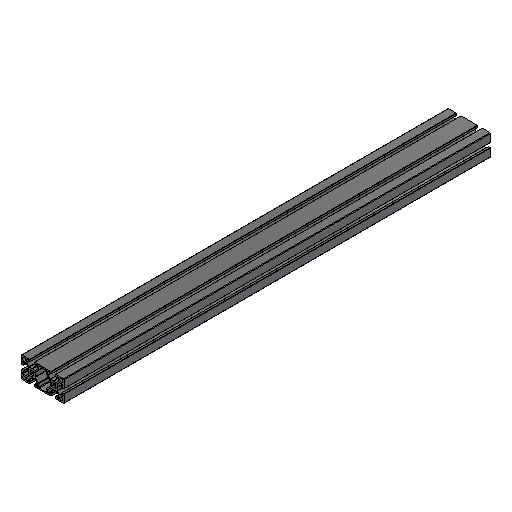
# Autodesk Inventor part: PROFILE
Saved by Autodesk Inventor 2022.5 (Build 265521000, 521)
## iProperties
Created: 2022-08-08
Part Number: PROFILE
Material: AL6061
Document SubType Name: Modeling
Designer: 박성규
Density: 2.7 g/cm^3
Description: 3
MAKER: DY PROFILE
DocNumber: DP 40X80-240L.ipt
Folder: 구매품\19. PIPE 형강류\AL PROFILE\DP TYPE\DP 40X80\
VDS_Category: 엔지니어링
Detail Description: Purchased products
Author: 최신영
Revision Number: B
Title: DP4080-802L
Autodesk Inventor part; units mm, degrees
ref_plane "YZ Plane" through (0, 0, 0) normal (1, 0, 0) x (0, 1, 0)
ref_plane "XZ Plane" through (0, 0, 0) normal (0, 1, 0) x (-1, 0, 0)
ref_plane "XY Plane" through (0, 0, 0) normal (0, 0, 1) x (1, 0, 0)
sketch "스케치3" plane through (0, 0, 0) normal (0, 0, 1) x (1, 0, 0)
  line L0 (0.0593, 17.8696) -> (6.8093, 17.8696)
  arc A0 (7.8093, 16.8696) -> (6.8093, 17.8696) centre (6.8093, 16.8696) ccw
  line L1 (7.8093, 16.8696) -> (7.8093, 10.9554)
  arc A1 (7.8093, 10.9554) -> (8.1022, 10.2483) centre (8.8093, 10.9554) ccw
  line L2 (8.1022, 10.2483) -> (14.2664, 4.0841)
  arc A2 (14.5593, 3.377) -> (14.2664, 4.0841) centre (13.5593, 3.377) ccw
  line L3 (14.5593, 3.377) -> (14.5593, -3.6377)
  arc A3 (14.2664, -4.3448) -> (14.5593, -3.6377) centre (13.5593, -3.6377) ccw
  line L4 (14.2664, -4.3448) -> (8.1022, -10.5091)
  arc A4 (8.1022, -10.5091) -> (7.8093, -11.2162) centre (8.8093, -11.2162) ccw
  line L5 (7.8093, -11.2162) -> (7.8093, -17.1304)
  arc A5 (6.8093, -18.1304) -> (7.8093, -17.1304) centre (6.8093, -17.1304) ccw
  line L6 (6.8093, -18.1304) -> (0.0593, -18.1304)
  line L7 (0.0593, -18.1304) -> (-6.6907, -18.1304)
  arc A6 (-7.6907, -17.1304) -> (-6.6907, -18.1304) centre (-6.6907, -17.1304) ccw
  line L8 (-7.6907, -17.1304) -> (-7.6907, -11.2162)
  arc A7 (-7.6907, -11.2162) -> (-7.9836, -10.5091) centre (-8.6907, -11.2162) ccw
  line L9 (-7.9836, -10.5091) -> (-14.1478, -4.3448)
  arc A8 (-14.4407, -3.6377) -> (-14.1478, -4.3448) centre (-13.4407, -3.6377) ccw
  line L10 (-14.4407, -3.6377) -> (-14.4407, 3.377)
  arc A9 (-14.1478, 4.0841) -> (-14.4407, 3.377) centre (-13.4407, 3.377) ccw
  line L11 (-14.1478, 4.0841) -> (-7.9836, 10.2483)
  arc A10 (-7.9836, 10.2483) -> (-7.6907, 10.9554) centre (-8.6907, 10.9554) ccw
  line L12 (-7.6907, 10.9554) -> (-7.6907, 16.8696)
  arc A11 (-6.6907, 17.8696) -> (-7.6907, 16.8696) centre (-6.6907, 16.8696) ccw
  line L13 (-6.6907, 17.8696) -> (0.0593, 17.8696)
  line L14 (39.0593, 19.8696) -> (24.7093, 19.8696)
  arc A12 (24.7093, 19.8696) -> (24.2093, 19.3696) centre (24.7093, 19.3696) ccw
  line L15 (24.2093, 19.3696) -> (24.2093, 16.1696)
  arc A13 (24.2093, 16.1696) -> (24.7093, 15.6696) centre (24.7093, 16.1696) ccw
  line L16 (24.7093, 15.6696) -> (26.6593, 15.6696)
  arc A14 (26.6593, 15.6696) -> (27.1593, 16.1696) centre (26.6593, 16.1696) ccw
  line L17 (27.1593, 16.1696) -> (27.1593, 17.3696)
  arc A15 (27.6593, 17.8696) -> (27.1593, 17.3696) centre (27.6593, 17.3696) ccw
  line L18 (27.6593, 17.8696) -> (29.8093, 17.8696)
  arc A16 (30.3093, 17.3696) -> (29.8093, 17.8696) centre (29.8093, 17.3696) ccw
  line L19 (30.3093, 17.3696) -> (30.3093, 12.061)
  arc A17 (30.1815, 11.7272) -> (30.3093, 12.061) centre (29.8093, 12.061) ccw
  line L20 (30.1815, 11.7272) -> (25.9734, 7.0358)
  arc A18 (25.6012, 6.8696) -> (25.9734, 7.0358) centre (25.6012, 7.3696) ccw
  line L21 (25.6012, 6.8696) -> (20.5593, 6.8696)
  line L22 (20.5593, 6.8696) -> (20.0593, 6.3696)
  line L23 (20.0593, 6.3696) -> (19.5593, 6.8696)
  line L24 (19.5593, 6.8696) -> (14.5174, 6.8696)
  arc A19 (14.1452, 7.0358) -> (14.5174, 6.8696) centre (14.5174, 7.3696) ccw
  line L25 (14.1452, 7.0358) -> (9.9371, 11.7272)
  arc A20 (9.8093, 12.061) -> (9.9371, 11.7272) centre (10.3093, 12.061) ccw
  line L26 (9.8093, 12.061) -> (9.8093, 17.3696)
  arc A21 (10.3093, 17.8696) -> (9.8093, 17.3696) centre (10.3093, 17.3696) ccw
  line L27 (10.3093, 17.8696) -> (12.4593, 17.8696)
  arc A22 (12.9593, 17.3696) -> (12.4593, 17.8696) centre (12.4593, 17.3696) ccw
  line L28 (12.9593, 17.3696) -> (12.9593, 16.1696)
  arc A23 (12.9593, 16.1696) -> (13.4593, 15.6696) centre (13.4593, 16.1696) ccw
  line L29 (13.4593, 15.6696) -> (15.4093, 15.6696)
  arc A24 (15.4093, 15.6696) -> (15.9093, 16.1696) centre (15.4093, 16.1696) ccw
  line L30 (15.9093, 16.1696) -> (15.9093, 19.3696)
  arc A25 (15.9093, 19.3696) -> (15.4093, 19.8696) centre (15.4093, 19.3696) ccw
  line L31 (15.4093, 19.8696) -> (-15.2907, 19.8696)
  arc A26 (-15.2907, 19.8696) -> (-15.7907, 19.3696) centre (-15.2907, 19.3696) ccw
  line L32 (-15.7907, 19.3696) -> (-15.7907, 16.1696)
  arc A27 (-15.7907, 16.1696) -> (-15.2907, 15.6696) centre (-15.2907, 16.1696) ccw
  line L33 (-15.2907, 15.6696) -> (-13.3407, 15.6696)
  arc A28 (-13.3407, 15.6696) -> (-12.8407, 16.1696) centre (-13.3407, 16.1696) ccw
  line L34 (-12.8407, 16.1696) -> (-12.8407, 17.3696)
  arc A29 (-12.3407, 17.8696) -> (-12.8407, 17.3696) centre (-12.3407, 17.3696) ccw
  line L35 (-12.3407, 17.8696) -> (-10.1907, 17.8696)
  arc A30 (-9.6907, 17.3696) -> (-10.1907, 17.8696) centre (-10.1907, 17.3696) ccw
  line L36 (-9.6907, 17.3696) -> (-9.6907, 11.8696)
  line L37 (-9.6907, 11.8696) -> (-14.1756, 6.8696)
  line L38 (-14.1756, 6.8696) -> (-19.4407, 6.8696)
  line L39 (-19.4407, 6.8696) -> (-19.9407, 6.3696)
  line L40 (-19.9407, 6.3696) -> (-20.4407, 6.8696)
  line L41 (-20.4407, 6.8696) -> (-25.4826, 6.8696)
  arc A31 (-25.8548, 7.0358) -> (-25.4826, 6.8696) centre (-25.4826, 7.3696) ccw
  line L42 (-25.8548, 7.0358) -> (-30.0629, 11.7272)
  arc A32 (-30.1907, 12.061) -> (-30.0629, 11.7272) centre (-29.6907, 12.061) ccw
  line L43 (-30.1907, 12.061) -> (-30.1907, 17.3696)
  arc A33 (-29.6907, 17.8696) -> (-30.1907, 17.3696) centre (-29.6907, 17.3696) ccw
  line L44 (-29.6907, 17.8696) -> (-27.5407, 17.8696)
  arc A34 (-27.0407, 17.3696) -> (-27.5407, 17.8696) centre (-27.5407, 17.3696) ccw
  line L45 (-27.0407, 17.3696) -> (-27.0407, 16.1696)
  arc A35 (-27.0407, 16.1696) -> (-26.5407, 15.6696) centre (-26.5407, 16.1696) ccw
  line L46 (-26.5407, 15.6696) -> (-24.5907, 15.6696)
  arc A36 (-24.5907, 15.6696) -> (-24.0907, 16.1696) centre (-24.5907, 16.1696) ccw
  line L47 (-24.0907, 16.1696) -> (-24.0907, 19.3696)
  arc A37 (-24.0907, 19.3696) -> (-24.5907, 19.8696) centre (-24.5907, 19.3696) ccw
  line L48 (-24.5907, 19.8696) -> (-38.9407, 19.8696)
  arc A38 (-38.9407, 19.8696) -> (-39.9407, 18.8696) centre (-38.9407, 18.8696) ccw
  line L49 (-39.9407, 18.8696) -> (-39.9407, 4.5196)
  arc A39 (-39.9407, 4.5196) -> (-39.4407, 4.0196) centre (-39.4407, 4.5196) ccw
  line L50 (-39.4407, 4.0196) -> (-36.2407, 4.0196)
  arc A40 (-36.2407, 4.0196) -> (-35.7407, 4.5196) centre (-36.2407, 4.5196) ccw
  line L51 (-35.7407, 4.5196) -> (-35.7407, 6.4696)
  arc A41 (-35.7407, 6.4696) -> (-36.2407, 6.9696) centre (-36.2407, 6.4696) ccw
  line L52 (-36.2407, 6.9696) -> (-37.4407, 6.9696)
  arc A42 (-37.9407, 7.4696) -> (-37.4407, 6.9696) centre (-37.4407, 7.4696) ccw
  line L53 (-37.9407, 7.4696) -> (-37.9407, 9.6196)
  arc A43 (-37.4407, 10.1196) -> (-37.9407, 9.6196) centre (-37.4407, 9.6196) ccw
  line L54 (-37.4407, 10.1196) -> (-32.1321, 10.1196)
  arc A44 (-31.7983, 9.9918) -> (-32.1321, 10.1196) centre (-32.1321, 9.6196) ccw
  line L55 (-31.7983, 9.9918) -> (-27.1069, 5.7837)
  arc A45 (-26.9407, 5.4115) -> (-27.1069, 5.7837) centre (-27.4407, 5.4115) ccw
  line L56 (-26.9407, 5.4115) -> (-26.9407, 0.3696)
  line L57 (-26.9407, 0.3696) -> (-26.4407, -0.1304)
  line L58 (-26.4407, -0.1304) -> (-26.9407, -0.6304)
  line L59 (-26.9407, -0.6304) -> (-26.9407, -5.6723)
  arc A46 (-27.1069, -6.0445) -> (-26.9407, -5.6723) centre (-27.4407, -5.6723) ccw
  line L60 (-27.1069, -6.0445) -> (-31.7983, -10.2526)
  arc A47 (-32.1321, -10.3804) -> (-31.7983, -10.2526) centre (-32.1321, -9.8804) ccw
  line L61 (-32.1321, -10.3804) -> (-37.4407, -10.3804)
  arc A48 (-37.9407, -9.8804) -> (-37.4407, -10.3804) centre (-37.4407, -9.8804) ccw
  line L62 (-37.9407, -9.8804) -> (-37.9407, -7.7304)
  arc A49 (-37.4407, -7.2304) -> (-37.9407, -7.7304) centre (-37.4407, -7.7304) ccw
  line L63 (-37.4407, -7.2304) -> (-36.2407, -7.2304)
  arc A50 (-36.2407, -7.2304) -> (-35.7407, -6.7304) centre (-36.2407, -6.7304) ccw
  line L64 (-35.7407, -6.7304) -> (-35.7407, -4.7804)
  arc A51 (-35.7407, -4.7804) -> (-36.2407, -4.2804) centre (-36.2407, -4.7804) ccw
  line L65 (-36.2407, -4.2804) -> (-39.4407, -4.2804)
  arc A52 (-39.4407, -4.2804) -> (-39.9407, -4.7804) centre (-39.4407, -4.7804) ccw
  line L66 (-39.9407, -4.7804) -> (-39.9407, -19.1304)
  arc A53 (-39.9407, -19.1304) -> (-38.9407, -20.1304) centre (-38.9407, -19.1304) ccw
  line L67 (-38.9407, -20.1304) -> (-24.5907, -20.1304)
  arc A54 (-24.5907, -20.1304) -> (-24.0907, -19.6304) centre (-24.5907, -19.6304) ccw
  line L68 (-24.0907, -19.6304) -> (-24.0907, -16.4304)
  arc A55 (-24.0907, -16.4304) -> (-24.5907, -15.9304) centre (-24.5907, -16.4304) ccw
  line L69 (-24.5907, -15.9304) -> (-26.5407, -15.9304)
  arc A56 (-26.5407, -15.9304) -> (-27.0407, -16.4304) centre (-26.5407, -16.4304) ccw
  line L70 (-27.0407, -16.4304) -> (-27.0407, -17.6304)
  arc A57 (-27.5407, -18.1304) -> (-27.0407, -17.6304) centre (-27.5407, -17.6304) ccw
  line L71 (-27.5407, -18.1304) -> (-29.6907, -18.1304)
  arc A58 (-30.1907, -17.6304) -> (-29.6907, -18.1304) centre (-29.6907, -17.6304) ccw
  line L72 (-30.1907, -17.6304) -> (-30.1907, -12.3218)
  arc A59 (-30.0629, -11.9879) -> (-30.1907, -12.3218) centre (-29.6907, -12.3218) ccw
  line L73 (-30.0629, -11.9879) -> (-25.8548, -7.2965)
  arc A60 (-25.4826, -7.1304) -> (-25.8548, -7.2965) centre (-25.4826, -7.6304) ccw
  line L74 (-25.4826, -7.1304) -> (-20.4407, -7.1304)
  line L75 (-20.4407, -7.1304) -> (-19.9407, -6.6304)
  line L76 (-19.9407, -6.6304) -> (-19.4407, -7.1304)
  line L77 (-19.4407, -7.1304) -> (-14.3988, -7.1304)
  arc A61 (-14.0266, -7.2965) -> (-14.3988, -7.1304) centre (-14.3988, -7.6304) ccw
  line L78 (-14.0266, -7.2965) -> (-9.8185, -11.9879)
  arc A62 (-9.6907, -12.3218) -> (-9.8185, -11.9879) centre (-10.1907, -12.3218) ccw
  line L79 (-9.6907, -12.3218) -> (-9.6907, -17.6304)
  arc A63 (-10.1907, -18.1304) -> (-9.6907, -17.6304) centre (-10.1907, -17.6304) ccw
  line L80 (-10.1907, -18.1304) -> (-12.3407, -18.1304)
  arc A64 (-12.8407, -17.6304) -> (-12.3407, -18.1304) centre (-12.3407, -17.6304) ccw
  line L81 (-12.8407, -17.6304) -> (-12.8407, -16.4304)
  arc A65 (-12.8407, -16.4304) -> (-13.3407, -15.9304) centre (-13.3407, -16.4304) ccw
  line L82 (-13.3407, -15.9304) -> (-15.2907, -15.9304)
  arc A66 (-15.2907, -15.9304) -> (-15.7907, -16.4304) centre (-15.2907, -16.4304) ccw
  line L83 (-15.7907, -16.4304) -> (-15.7907, -19.6304)
  arc A67 (-15.7907, -19.6304) -> (-15.2907, -20.1304) centre (-15.2907, -19.6304) ccw
  line L84 (-15.2907, -20.1304) -> (0.0593, -20.1304)
  line L85 (0.0593, -20.1304) -> (15.4093, -20.1304)
  arc A68 (15.4093, -20.1304) -> (15.9093, -19.6304) centre (15.4093, -19.6304) ccw
  line L86 (15.9093, -19.6304) -> (15.9093, -16.4304)
  arc A69 (15.9093, -16.4304) -> (15.4093, -15.9304) centre (15.4093, -16.4304) ccw
  line L87 (15.4093, -15.9304) -> (13.4593, -15.9304)
  arc A70 (13.4593, -15.9304) -> (12.9593, -16.4304) centre (13.4593, -16.4304) ccw
  line L88 (12.9593, -16.4304) -> (12.9593, -17.6304)
  arc A71 (12.4593, -18.1304) -> (12.9593, -17.6304) centre (12.4593, -17.6304) ccw
  line L89 (12.4593, -18.1304) -> (10.3093, -18.1304)
  arc A72 (9.8093, -17.6304) -> (10.3093, -18.1304) centre (10.3093, -17.6304) ccw
  line L90 (9.8093, -17.6304) -> (9.8093, -12.3218)
  arc A73 (9.9371, -11.9879) -> (9.8093, -12.3218) centre (10.3093, -12.3218) ccw
  line L91 (9.9371, -11.9879) -> (14.1452, -7.2965)
  arc A74 (14.5174, -7.1304) -> (14.1452, -7.2965) centre (14.5174, -7.6304) ccw
  line L92 (14.5174, -7.1304) -> (19.5593, -7.1304)
  line L93 (19.5593, -7.1304) -> (20.0593, -6.6304)
  line L94 (20.0593, -6.6304) -> (20.5593, -7.1304)
  line L95 (20.5593, -7.1304) -> (25.6012, -7.1304)
  arc A75 (25.9734, -7.2965) -> (25.6012, -7.1304) centre (25.6012, -7.6304) ccw
  line L96 (25.9734, -7.2965) -> (30.1815, -11.9879)
  arc A76 (30.3093, -12.3218) -> (30.1815, -11.9879) centre (29.8093, -12.3218) ccw
  line L97 (30.3093, -12.3218) -> (30.3093, -17.6304)
  arc A77 (29.8093, -18.1304) -> (30.3093, -17.6304) centre (29.8093, -17.6304) ccw
  line L98 (29.8093, -18.1304) -> (27.6593, -18.1304)
  arc A78 (27.1593, -17.6304) -> (27.6593, -18.1304) centre (27.6593, -17.6304) ccw
  line L99 (27.1593, -17.6304) -> (27.1593, -16.4304)
  arc A79 (27.1593, -16.4304) -> (26.6593, -15.9304) centre (26.6593, -16.4304) ccw
  line L100 (26.6593, -15.9304) -> (24.7093, -15.9304)
  arc A80 (24.7093, -15.9304) -> (24.2093, -16.4304) centre (24.7093, -16.4304) ccw
  line L101 (24.2093, -16.4304) -> (24.2093, -19.6304)
  arc A81 (24.2093, -19.6304) -> (24.7093, -20.1304) centre (24.7093, -19.6304) ccw
  line L102 (24.7093, -20.1304) -> (39.0593, -20.1304)
  arc A82 (39.0593, -20.1304) -> (40.0593, -19.1304) centre (39.0593, -19.1304) ccw
  line L103 (40.0593, -19.1304) -> (40.0593, -4.7804)
  arc A83 (40.0593, -4.7804) -> (39.5593, -4.2804) centre (39.5593, -4.7804) ccw
  line L104 (39.5593, -4.2804) -> (36.3593, -4.2804)
  arc A84 (36.3593, -4.2804) -> (35.8593, -4.7804) centre (36.3593, -4.7804) ccw
  line L105 (35.8593, -4.7804) -> (35.8593, -6.7304)
  arc A85 (35.8593, -6.7304) -> (36.3593, -7.2304) centre (36.3593, -6.7304) ccw
  line L106 (36.3593, -7.2304) -> (37.5593, -7.2304)
  arc A86 (38.0593, -7.7304) -> (37.5593, -7.2304) centre (37.5593, -7.7304) ccw
  line L107 (38.0593, -7.7304) -> (38.0593, -9.8804)
  arc A87 (37.5593, -10.3804) -> (38.0593, -9.8804) centre (37.5593, -9.8804) ccw
  line L108 (37.5593, -10.3804) -> (32.2507, -10.3804)
  arc A88 (31.9168, -10.2526) -> (32.2507, -10.3804) centre (32.2507, -9.8804) ccw
  line L109 (31.9168, -10.2526) -> (27.2254, -6.0445)
  arc A89 (27.0593, -5.6723) -> (27.2254, -6.0445) centre (27.5593, -5.6723) ccw
  line L110 (27.0593, -5.6723) -> (27.0593, -0.6304)
  line L111 (27.0593, -0.6304) -> (26.5593, -0.1304)
  line L112 (26.5593, -0.1304) -> (27.0593, 0.3696)
  line L113 (27.0593, 0.3696) -> (27.0593, 5.4115)
  arc A90 (27.2254, 5.7837) -> (27.0593, 5.4115) centre (27.5593, 5.4115) ccw
  line L114 (27.2254, 5.7837) -> (31.9168, 9.9918)
  arc A91 (32.2507, 10.1196) -> (31.9168, 9.9918) centre (32.2507, 9.6196) ccw
  line L115 (32.2507, 10.1196) -> (37.5593, 10.1196)
  arc A92 (38.0593, 9.6196) -> (37.5593, 10.1196) centre (37.5593, 9.6196) ccw
  line L116 (38.0593, 9.6196) -> (38.0593, 7.4696)
  arc A93 (37.5593, 6.9696) -> (38.0593, 7.4696) centre (37.5593, 7.4696) ccw
  line L117 (37.5593, 6.9696) -> (36.3593, 6.9696)
  arc A94 (36.3593, 6.9696) -> (35.8593, 6.4696) centre (36.3593, 6.4696) ccw
  line L118 (35.8593, 6.4696) -> (35.8593, 4.5196)
  arc A95 (35.8593, 4.5196) -> (36.3593, 4.0196) centre (36.3593, 4.5196) ccw
  line L119 (36.3593, 4.0196) -> (39.5593, 4.0196)
  arc A96 (39.5593, 4.0196) -> (40.0593, 4.5196) centre (39.5593, 4.5196) ccw
  line L120 (40.0593, 4.5196) -> (40.0593, 18.8696)
  arc A97 (40.0593, 18.8696) -> (39.0593, 19.8696) centre (39.0593, 18.8696) ccw
  circle A98 centre (-34.9407, 14.8696) radius 3
  arc A99 (-16.3285, 3.1805) -> (-16.6298, 3.4818) centre (-19.9407, -0.1304) ccw
  arc A100 (-16.6298, 3.4818) -> (-17.0447, 3.4728) centre (-16.8325, 3.2607) ccw
  line L121 (-17.0447, 3.4728) -> (-17.7399, 2.7776)
  arc A101 (-18.1132, 2.7367) -> (-17.7399, 2.7776) centre (-17.952, 2.9897) ccw
  arc A102 (-18.1132, 2.7367) -> (-21.7682, 2.7367) centre (-19.9407, -0.1304) ccw
  arc A103 (-22.1416, 2.7776) -> (-21.7682, 2.7367) centre (-21.9294, 2.9897) ccw
  line L122 (-22.1416, 2.7776) -> (-22.8368, 3.4728)
  arc A104 (-22.8368, 3.4728) -> (-23.2516, 3.4818) centre (-23.0489, 3.2607) ccw
  arc A105 (-23.2516, 3.4818) -> (-23.5529, 3.1805) centre (-19.9407, -0.1304) ccw
  arc A106 (-23.5529, 3.1805) -> (-23.5439, 2.7657) centre (-23.3318, 2.9778) ccw
  line L123 (-23.5439, 2.7657) -> (-22.8487, 2.0705)
  arc A107 (-22.8078, 1.6971) -> (-22.8487, 2.0705) centre (-23.0608, 1.8583) ccw
  arc A108 (-22.8078, 1.6971) -> (-22.8078, -1.9578) centre (-19.9407, -0.1304) ccw
  arc A109 (-22.8487, -2.3312) -> (-22.8078, -1.9578) centre (-23.0608, -2.1191) ccw
  line L124 (-22.8487, -2.3312) -> (-23.5439, -3.0264)
  arc A110 (-23.5439, -3.0264) -> (-23.5529, -3.4413) centre (-23.3318, -3.2386) ccw
  arc A111 (-23.5529, -3.4413) -> (-23.2516, -3.7426) centre (-19.9407, -0.1304) ccw
  arc A112 (-23.2516, -3.7426) -> (-22.8368, -3.7335) centre (-23.0489, -3.5214) ccw
  line L125 (-22.8368, -3.7335) -> (-22.1416, -3.0383)
  arc A113 (-21.7682, -2.9975) -> (-22.1416, -3.0383) centre (-21.9294, -3.2505) ccw
  arc A114 (-21.7682, -2.9975) -> (-18.1132, -2.9975) centre (-19.9407, -0.1304) ccw
  arc A115 (-17.7399, -3.0383) -> (-18.1132, -2.9975) centre (-17.952, -3.2505) ccw
  line L126 (-17.7399, -3.0383) -> (-17.0447, -3.7335)
  arc A116 (-17.0447, -3.7335) -> (-16.6298, -3.7426) centre (-16.8325, -3.5214) ccw
  arc A117 (-16.6298, -3.7426) -> (-16.3285, -3.4413) centre (-19.9407, -0.1304) ccw
  arc A118 (-16.3285, -3.4413) -> (-16.3376, -3.0264) centre (-16.5497, -3.2386) ccw
  line L127 (-16.3376, -3.0264) -> (-17.0328, -2.3312)
  arc A119 (-17.0736, -1.9578) -> (-17.0328, -2.3312) centre (-16.8206, -2.1191) ccw
  arc A120 (-17.0736, -1.9578) -> (-17.0736, 1.6971) centre (-19.9407, -0.1304) ccw
  arc A121 (-17.0328, 2.0705) -> (-17.0736, 1.6971) centre (-16.8206, 1.8583) ccw
  line L128 (-17.0328, 2.0705) -> (-16.3376, 2.7657)
  arc A122 (-16.3376, 2.7657) -> (-16.3285, 3.1805) centre (-16.5497, 2.9778) ccw
  circle A123 centre (-34.9407, -15.1304) radius 3
  circle A124 centre (35.0593, 14.8696) radius 3
  arc A125 (16.7484, 3.4818) -> (16.4471, 3.1805) centre (20.0593, -0.1304) ccw
  arc A126 (17.1632, 3.4728) -> (16.7484, 3.4818) centre (16.9511, 3.2607) ccw
  line L129 (17.1632, 3.4728) -> (17.8584, 2.7776)
  arc A127 (17.8584, 2.7776) -> (18.2318, 2.7367) centre (18.0706, 2.9897) ccw
  arc A128 (21.8868, 2.7367) -> (18.2318, 2.7367) centre (20.0593, -0.1304) ccw
  arc A129 (21.8868, 2.7367) -> (22.2601, 2.7776) centre (22.048, 2.9897) ccw
  line L130 (22.2601, 2.7776) -> (22.9553, 3.4728)
  arc A130 (23.3702, 3.4818) -> (22.9553, 3.4728) centre (23.1675, 3.2607) ccw
  arc A131 (23.6715, 3.1805) -> (23.3702, 3.4818) centre (20.0593, -0.1304) ccw
  arc A132 (23.6624, 2.7657) -> (23.6715, 3.1805) centre (23.4503, 2.9778) ccw
  line L131 (23.6624, 2.7657) -> (22.9672, 2.0705)
  arc A133 (22.9672, 2.0705) -> (22.9264, 1.6971) centre (23.1794, 1.8583) ccw
  arc A134 (22.9264, -1.9578) -> (22.9264, 1.6971) centre (20.0593, -0.1304) ccw
  arc A135 (22.9264, -1.9578) -> (22.9672, -2.3312) centre (23.1794, -2.1191) ccw
  line L132 (22.9672, -2.3312) -> (23.6624, -3.0264)
  arc A136 (23.6715, -3.4413) -> (23.6624, -3.0264) centre (23.4503, -3.2386) ccw
  arc A137 (23.3702, -3.7426) -> (23.6715, -3.4413) centre (20.0593, -0.1304) ccw
  arc A138 (22.9553, -3.7335) -> (23.3702, -3.7426) centre (23.1675, -3.5214) ccw
  line L133 (22.9553, -3.7335) -> (22.2601, -3.0383)
  arc A139 (22.2601, -3.0383) -> (21.8868, -2.9975) centre (22.048, -3.2505) ccw
  arc A140 (18.2318, -2.9975) -> (21.8868, -2.9975) centre (20.0593, -0.1304) ccw
  arc A141 (18.2318, -2.9975) -> (17.8584, -3.0383) centre (18.0706, -3.2505) ccw
  line L134 (17.8584, -3.0383) -> (17.1632, -3.7335)
  arc A142 (16.7484, -3.7426) -> (17.1632, -3.7335) centre (16.9511, -3.5214) ccw
  arc A143 (16.4471, -3.4413) -> (16.7484, -3.7426) centre (20.0593, -0.1304) ccw
  arc A144 (16.4561, -3.0264) -> (16.4471, -3.4413) centre (16.6682, -3.2386) ccw
  line L135 (16.4561, -3.0264) -> (17.1513, -2.3312)
  arc A145 (17.1513, -2.3312) -> (17.1922, -1.9578) centre (16.9392, -2.1191) ccw
  arc A146 (17.1922, 1.6971) -> (17.1922, -1.9578) centre (20.0593, -0.1304) ccw
  arc A147 (17.1922, 1.6971) -> (17.1513, 2.0705) centre (16.9392, 1.8583) ccw
  line L136 (17.1513, 2.0705) -> (16.4561, 2.7657)
  arc A148 (16.4471, 3.1805) -> (16.4561, 2.7657) centre (16.6682, 2.9778) ccw
  circle A149 centre (35.0593, -15.1304) radius 3
  constraints: 292 point on circle, 274 end point, 150 centre point
extrude "돌출1" add sketch "스케치3" along normal mid plane 802
